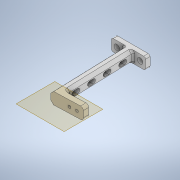
# Autodesk Inventor part: 2200_support_3
Saved by Autodesk Inventor 2020 (Build 240168000, 168)
## iProperties
Created: 2019-10-23
Part Number: 2200_support_3
Material: Generic
Document SubType Name: Modeling
Designer: psrob
Density: 1 g/cm^3
Appearance: Default
Author: psrob
Autodesk Inventor part; units mm, degrees
ref_plane "YZ Plane" through (0, 0, 0) normal (1, 0, 0) x (0, 1, 0)
ref_plane "XZ Plane" through (0, 0, 0) normal (0, 1, 0) x (-1, 0, 0)
ref_plane "XY Plane" through (0, 0, 0) normal (0, 0, 1) x (1, 0, 0)
ref_plane "Work Plane1" through (13.3856, -75.691, 8.7894) normal (0, 1, 0) x (-1, 0, 0)
sketch "Sketch1" plane through (13.3856, -75.691, 8.7894) normal (0, 1, 0) x (-1, 0, 0)
  line L0 (-15.3087, 11.6251) -> (21.19, 11.8493) projected
  arc A0 (24.2084, 8.8678) -> (21.19, 11.8493) centre (21.2084, 8.8494) ccw projected
  line L1 (24.2084, 8.8678) -> (24.2713, -1.3839) projected
  arc A1 (21.2898, -4.4023) -> (24.2713, -1.3839) centre (21.2714, -1.4024) ccw projected
  line L2 (21.2898, -4.4023) -> (-15.1011, -4.6259) projected
  arc A2 (-15.1011, -4.6259) -> (-19.1843, -8.625) centre (-15.1843, -8.625) ccw projected
  line L3 (-19.1843, -8.625) -> (-19.1843, -17.625) projected
  arc A3 (-19.1843, -17.625) -> (-17.1843, -19.625) centre (-17.1843, -17.625) ccw projected
  line L4 (-17.1843, -19.625) -> (-13.1843, -19.625) projected
  arc A4 (-13.1843, -19.625) -> (-11.1843, -17.625) centre (-13.1843, -17.625) ccw projected
  line L5 (-11.1843, -17.625) -> (-11.1843, -14.4296) projected
  arc A5 (-9.2505, -12.4307) -> (-11.1843, -14.4296) centre (-9.1843, -14.4296) ccw projected
  line L6 (-9.2505, -12.4307) -> (26.4128, -11.25) projected
  arc A6 (26.4128, -11.25) -> (29.3135, -8.2332) centre (26.3136, -8.2516) ccw projected
  line L7 (29.3135, -8.2332) -> (29.1689, 15.306) projected
  arc A7 (29.1689, 15.306) -> (26.2655, 18.286) centre (26.169, 15.2876) ccw projected
  line L8 (26.2655, 18.286) -> (-15.0761, 19.6167) projected
  arc A8 (-15.0761, 19.6167) -> (-15.3087, 11.6251) centre (-15.3333, 15.625) ccw projected
  circle A9 centre (-15.1843, -8.625) radius 1.5 projected
  circle A10 centre (-15.3333, 15.625) radius 1.5 projected
  circle A11 centre (-15.1843, -15.625) radius 1.5 projected
  line L9 (-9.2505, -12.4307) -> (25.7303, -11.2726)
  line L10 (90.6667, -101.625) -> (-109.3333, -101.625) projected
  line L11 (25.7303, -11.2726) -> (28.7218, -101.625)
  line L12 (28.7218, -101.625) -> (18.7218, -101.625)
  line L13 (18.7218, -101.625) -> (16.0084, -19.6699)
  line L14 (16.0084, -19.6699) -> (-8.9779, -20.4972)
  line L15 (-9.2505, -12.4307) -> (-8.9779, -20.4972)
  point P0 (13.3856, -8.7894)
  dimension "d0" = 35
  dimension "d1" = 10
  dimension "d2" = 82
  dimension "d3" = 25
  constraints: 12 end point, 3 point on line, 2 parallel, 1 perpendicular
  measures "d0" distance of L6.start L9.end
  measures "d1" distance of L11.end L12.end
  measures "d2" distance of L12.end L13.end
  measures "d3" distance of L13.end L14.end
ref_plane "Work Plane2" through (-15.928, -88.691, -10.8356) normal (0, -1, 0) x (1, 0, 0)
extrude "Extrusion1" add sketch "Sketch1" against normal up to surface (13 mm away) contours L11 L10 L13 L14 L15 L6
sketch "Sketch2" plane through (-2.6228, -88.691, -10.8805) normal (-0.0330906, 0, -0.9994524) x (-0.9994524, 0, 0.0330906)
  circle A0 centre (-18.0055, 6.5) radius 1.5 projected
  circle A1 centre (-10.0055, 6.5) radius 1.5 projected
  point P0 (-2.2613, 88.691)
extrude "Extrusion2" cut sketch "Sketch2" against normal blind 10
sketch "Sketch3" plane through (13.3856, -75.691, 8.7894) normal (0, 1, 0) x (1, 0, 0)
  line L0 (109.3333, 100.625) -> (-90.6667, 100.625) projected
  line L1 (8.9779, 20.4972) -> (-16.0084, 19.6699) projected
  line L2 (-16.0084, 19.6699) -> (-18.7218, 101.625) projected
  line L3 (-18.7218, 101.625) -> (-28.7218, 101.625) projected
  line L4 (-28.7218, 101.625) -> (-25.7303, 11.2726) projected
  line L5 (-25.7303, 11.2726) -> (9.2505, 12.4307) projected
  line L6 (9.2505, 12.4307) -> (8.9779, 20.4972) projected
  point P0 (-13.3856, 8.7894)
  point P1 (-28.6887, 100.625)
  point P2 (-18.6887, 100.625)
extrude "Extrusion3" cut sketch "Sketch3" against normal blind 18 contours L0 L4 L3 L2
sketch "Sketch4" plane through (13.3856, -75.691, 8.7894) normal (0, 1, 0) x (1, 0, 0)
  line L0 (-18.6887, 100.625) -> (-28.6887, 100.625) projected
  line L1 (-28.6887, 100.625) -> (-25.7303, 11.2726) projected
  line L2 (-25.7303, 11.2726) -> (9.2505, 12.4307) projected
  line L3 (9.2505, 12.4307) -> (8.9779, 20.4972) projected
  line L4 (8.9779, 20.4972) -> (-16.0084, 19.6699) projected
  line L5 (-16.0084, 19.6699) -> (-18.6887, 100.625) projected
  line L6 (109.3333, 100.625) -> (-90.6667, 100.625) projected
  line L7 (-28.6887, 100.625) -> (-42.6887, 100.625)
  line L8 (-18.6887, 100.625) -> (-28.6887, 100.625) projected
  line L9 (-18.6887, 100.625) -> (-4.6887, 100.625)
  line L10 (-4.6887, 100.625) -> (-4.6887, 95.625)
  line L11 (-4.6887, 95.625) -> (-18.5231, 95.625)
  line L12 (-28.5231, 95.625) -> (-42.6887, 95.625)
  line L13 (-42.6887, 95.625) -> (-42.6887, 100.625)
  point P0 (-13.3856, 8.7894)
  dimension "d10" = 14
  dimension "d11" = 14
  dimension "d12" = 5
  constraints: 12 end point, 6 point on line, 2 perpendicular, 1 vertical
  measures "d10" distance of L0.end L7.end
  measures "d11" distance of L0.start L9.end
  measures "d12" distance of L9.end L10.end
extrude "Extrusion4" add sketch "Sketch4" against normal up to surface (13 mm away) contours L6 L10 L11 L5 | L1 L12 L13 L6
sketch "Sketch5" plane through (-5.1376, -75.691, -86.8356) normal (0, 0, 1) x (1, 0, 0)
  line L0 (-24.1655, -13) -> (-10, -13) projected
  line L1 (-10, 0) -> (-10, -13) projected
  line L2 (-24.1655, 0) -> (-10, 0) projected
  line L3 (-24.1655, 0) -> (-24.1655, -13) projected
  line L4 (0, -13) -> (13.8345, -13) projected
  line L5 (13.8345, 0) -> (13.8345, -13) projected
  line L6 (0, 0) -> (13.8345, 0) projected
  line L7 (0, -13) -> (0, 0) projected
  line L8 (-24.1655, -6.5) -> (-18.1655, -6.5)
  circle A0 centre (-18.1655, -6.5) radius 3
  line L9 (13.8345, -6.5) -> (7.8345, -6.5)
  circle A1 centre (7.8345, -6.5) radius 3
  point P0 (5.1376, 75.691)
  dimension "d15" = 6
  dimension "d16" = 6
  dimension "d17" = 6
  dimension "d18" = 6
  constraints: 4 end point, 2 centre point, 2 coincident, 2 horizontal, 2 midpoint
  measures "d15" distance of L8.start L8.end
  measures "d16" diameter of A0
  measures "d17" distance of L9.start L9.end
  measures "d18" diameter of A1
extrude "Extrusion5" cut sketch "Sketch5" against normal blind 18 contours A0 | A1
thicken "Thicken1" operation add thickness 2 both sides no extend neighbours yes toward (0.0330906, 0, 0.9994524) faces at (9.0995, -77.3613, -11.2686)
chamfer "Chamfer1" distance 3 angle 45 4 edges at (-3.8471, -88.691, -47.8586) (-13.7412, -88.691, -44.6594) (-3.8471, -75.691, -47.8586) (-13.7412, -75.691, -44.6594)
fillet "Fillet1" radius 2 6 edges at (-13.6367, -77.191, -86.8356) (-15.1376, -82.191, -86.8356) (-13.6367, -87.191, -86.8356) (-6.6384, -77.191, -86.8356) (-5.1376, -82.191, -86.8356) (-6.6384, -87.191, -86.8356)
fillet "Fillet2" radius 2 4 edges at (8.6969, -75.691, -89.3356) (8.6969, -88.691, -89.3356) (-29.3031, -75.691, -89.3356) (-29.3031, -88.691, -89.3356)
fillet "Fillet3" radius 5 3 edges at (-4.0558, -87.191, -8.832) (-2.5566, -82.191, -8.8816) (-4.0558, -77.191, -8.832)
fillet "Fillet4" radius 3 2 edges at (22.5336, -88.691, -6.6751) (22.5336, -75.691, -6.6751)
sketch "Sketch6" plane through (-12.3448, -85.691, -2.4832) normal (-0.9994524, 0, 0.0330906) x (0.0330906, 0, 0.9994524)
  line L0 (-82.4638, -0.0001) -> (-82.4638, 7.0001) projected
  ellipse E0 centre (-82.3976, -2.8284) end of major axis (-82.4912, -0.0008) minor radius 2 (-82.4444, 0) -> (-82.4638, -0.0001) ccw projected
  line L1 (0, 0) -> (-82.4444, 0) projected
  line L2 (0, 7) -> (0, 0) projected
  line L3 (-82.4444, 7) -> (0, 7) projected
  ellipse E1 centre (-82.3976, 9.8284) end of major axis (-82.4912, 7.0008) minor radius 2 (-82.4638, 7.0001) -> (-82.4444, 7) ccw projected
  line L4 (0, 7) -> (0, 0) projected
  line L5 (0, 3.5) -> (-18, 3.5)
  line L6 (-16, 3.5) -> (-20, 3.5) construction
  line L7 (-16, 6) -> (-20, 6)
  line L8 (-20, 1) -> (-16, 1)
  arc A0 (-16, 1) -> (-16, 6) centre (-16, 3.5) ccw
  arc A1 (-20, 6) -> (-20, 1) centre (-20, 3.5) ccw
  arc A2 (-38, 6) -> (-38, 1) centre (-38, 3.5) ccw
  line L9 (-34, 6) -> (-38, 6)
  line L10 (-38, 1) -> (-34, 1)
  arc A3 (-34, 1) -> (-34, 6) centre (-34, 3.5) ccw
  arc A4 (-56, 6) -> (-56, 1) centre (-56, 3.5) ccw
  line L11 (-52, 6) -> (-56, 6)
  line L12 (-56, 1) -> (-52, 1)
  arc A5 (-52, 1) -> (-52, 6) centre (-52, 3.5) ccw
  arc A6 (-74, 6) -> (-74, 1) centre (-74, 3.5) ccw
  line L13 (-70, 6) -> (-74, 6)
  line L14 (-74, 1) -> (-70, 1)
  arc A7 (-70, 1) -> (-70, 6) centre (-70, 3.5) ccw
  point P0 (2.8903, 85.691)
  dimension "d30" = 18
  dimension "d31" = 2
  dimension "d32" = 5
  dimension "d35" = 18
  constraints: 22 end point, 16 point on circle, 8 centre point, 4 tangent, 3 horizontal, 2 midpoint, 1 parallel, 32 other
  measures "d30" distance of L5.start L5.end
  measures "d31" distance of L5.end L6.end
  measures "d32" diameter of A1
  measures "d35" distance of L6.end A2.centre
extrude "Extrusion6" cut sketch "Sketch6" against normal blind 18 contours A0 L8 A1 L7 | L9 A3 L10 A2 | L11 A5 L12 A4 | L13 A7 L14 A6
body "Solid1"
